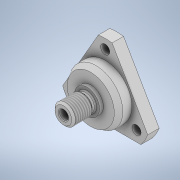
# Autodesk Inventor part: Деталь1
Saved by Autodesk Inventor 2021 (Build 250183000, 183)
## iProperties
Created: 2020-05-29
Part Number: Деталь1
Material: Типовые
Document SubType Name: Modeling
Designer: 2000
Density: 1 g/cm^3
Appearance: По умолчанию
Mass: 147.285 g
Surface Area: 309.668 cm^2
Volume: 147.285 cm^3
Author: 2000
Autodesk Inventor part; units mm, degrees
ref_plane "YZ Plane" through (0, 0, 0) normal (1, 0, 0) x (0, 1, 0)
ref_plane "XZ Plane" through (0, 0, 0) normal (0, 1, 0) x (-1, 0, 0)
ref_plane "XY Plane" through (0, 0, 0) normal (0, 0, 1) x (1, 0, 0)
sketch "Эскиз1" plane through (0, 0, 0) normal (0, 0, 1) x (1, 0, 0)
  line L0 (-9.0572, 59.3125) -> (-55.8947, -21.8125)
  line L1 (-46.8375, -37.5) -> (46.8375, -37.5)
  line L2 (9.0572, 59.3125) -> (55.8947, -21.8125)
  arc A0 (9.0572, 59.3125) -> (-9.0572, 59.3125) centre (0, 0) ccw
  arc A1 (-55.8947, -21.8125) -> (-46.8375, -37.5) centre (0, 0) ccw
  arc A2 (46.8375, -37.5) -> (55.8947, -21.8125) centre (0, 0) ccw
  circle A3 centre (0, 47.5) radius 6
  circle A4 centre (41.1362, -23.75) radius 6
  circle A5 centre (-41.1362, -23.75) radius 6
  point P0 (51.9615, -30)
  dimension "d3" = 12
  dimension "d4" = 12
  dimension "d5" = 12
  dimension "d7" = 47.5
  dimension "d8" = 41.1362
  dimension "d9" = 41.1362
  dimension "d10" = 13.75
  dimension "d11" = 13.75
  dimension "d12" = 13.75
  constraints: 7 point on circle, 6 centre point, 6 end point, 2 horizontal, 5 other
  measures "d3" diameter of A3
  measures "d4" diameter of A4
  measures "d5" diameter of A5
  measures "d7" distance of point (0, 0) A3.centre
  measures "d8" horizontal distance of point (0, 0) A4.centre
  measures "d9" horizontal distance of point (0, 0) A5.centre
  measures "d10" distance from line of L0 A3.centre
  measures "d11" distance from line of L2 A4.centre
  measures "d12" distance from line of L1 A5.centre
extrude "Выдавливание1" add sketch "Эскиз1" along normal blind 15
sketch "Эскиз2" plane through (0, 0, 15) normal (0, 0, 1) x (1, 0, 0)
  circle A0 centre (0, 0) radius 35
  dimension "d15" = 70
  constraints: 1 centre point, 1 coincident
  measures "d15" diameter of A0
extrude "Выдавливание2" add sketch "Эскиз2" along normal blind 19
sketch "Эскиз4" plane through (0, 0, 0) normal (0, 1, 0) x (-1, 0, 0)
  line L0 (35, 34) -> (-35, 34) projected
  line L1 (30.9218, 34) -> (35, 26.9363)
  line L2 (35, 15) -> (35, 34) projected
  line L3 (30.9218, 34) -> (35, 34)
  line L4 (0, -6.8) -> (0, 40.8) projected
  point P0 (0, 0)
  dimension "d21" = 30
  constraints: 4 end point, 2 point on line, 1 collinear
  measures "d21" angle of L2 L1
revolve "Вращение1" cut sketch "Эскиз4" angle 360 about axis through (0, 0, -10) along (0, 0, 1)
sketch "Эскиз5" plane through (0, 0, 34) normal (0, 0, 1) x (1, 0, 0)
  circle A0 centre (0, 0) radius 16.5
  dimension "d23" = 33
  constraints: 1 centre point, 1 coincident
  measures "d23" diameter of A0
extrude "Выдавливание3" add sketch "Эскиз5" along normal blind 5
sketch "Эскиз6" plane through (0, 0, 39) normal (0, 0, 1) x (1, 0, 0)
  circle A0 centre (0, 0) radius 11.25
  dimension "d26" = 22.5
  constraints: 1 centre point, 1 coincident
  measures "d26" diameter of A0
extrude "Выдавливание4" add sketch "Эскиз6" along normal blind 7
sketch "Эскиз7" plane through (0, 0, 46) normal (0, 0, 1) x (1, 0, 0)
  circle A0 centre (0, 0) radius 13.5
  dimension "d29" = 27
  constraints: 1 centre point, 1 coincident
  measures "d29" diameter of A0
extrude "Выдавливание5" add sketch "Эскиз7" along normal blind 24
sketch "Эскиз8" plane through (0, 0, 0) normal (0, 0, -1) x (-1, 0, 0)
  circle A0 centre (0, 0) radius 27
  dimension "d32" = 54
  constraints: 1 centre point, 1 coincident
  measures "d32" diameter of A0
extrude "Выдавливание6" cut sketch "Эскиз8" against normal blind 10
sketch "Эскиз15" plane through (0, 0, 10) normal (0, 0, -1) x (-1, 0, 0)
  circle A0 centre (0, 0) radius 14
  dimension "d54" = 28
  constraints: 1 centre point, 1 coincident
  measures "d54" diameter of A0
extrude "Выдавливание11" cut sketch "Эскиз15" against normal blind 21
chamfer "Фаска1" distance 6 angle 45 1 edges at (14, 0, 10)
sketch "Эскиз16" plane through (0, 0, 31) normal (0, 0, -1) x (-1, 0, 0)
  circle A0 centre (0, 0) radius 6
  dimension "d60" = 12
  constraints: 1 centre point, 1 coincident
  measures "d60" diameter of A0
extrude "Выдавливание12" cut sketch "Эскиз16" against normal blind 39
thread "Резьба1" size "M27x3" class "6g" standard "ANSI Metric M Profile" full length
fillet "Сопряжение1" radius 1.6 1 edges at (-11.25, 0, 39)
chamfer "Фаска2" distance 2.25 angle 45 1 edges at (-11.25, 0, 46)
fillet "Сопряжение2" radius 1 1 edges at (-11.25, 0, 43.7501)
chamfer "Фаска3" distance 2.5 angle 45 1 edges at (-13.5, 0, 70)
chamfer "Фаска4" distance 1 angle 45 1 edges at (6, 0, 70)
